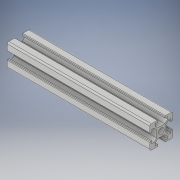
# Autodesk Inventor part: 2020-125mm
Saved by Autodesk Inventor 2019 (Build 230136000, 136)
## iProperties
Created: 2019-04-21
Part Number: 2020-125mm
Material: Generic
Document SubType Name: Modeling
Designer: Alex Jones
Density: 1 g/cm^3
Appearance: Default
Author: Alex Jones
Autodesk Inventor part; units mm, degrees
ref_plane "YZ Plane" through (0, 0, 0) normal (1, 0, 0) x (0, 1, 0)
ref_plane "XZ Plane" through (0, 0, 0) normal (0, 1, 0) x (-1, 0, 0)
ref_plane "XY Plane" through (0, 0, 0) normal (0, 0, 1) x (1, 0, 0)
sketch "Sketch1" plane through (0, 0, 0) normal (1, 0, 0) x (0, 1, 0)
  circle A0 centre (0, 0) radius 2.5
  line L0 (0, 0) -> (10, 0)
  line L1 (10, -10) -> (10, -3.6)
  line L2 (10, -3.6) -> (9.5, -3.1)
  line L3 (9.5, -3.1) -> (8.4, -3.1)
  line L4 (8.4, -3.1) -> (8.4, -5.5)
  line L5 (-3.134, 4.1) -> (3.134, 4.1)
  line L6 (4.1, 3.134) -> (4.1, -3.134)
  line L7 (3.134, -4.1) -> (-3.134, -4.1)
  line L8 (-4.1, -3.134) -> (-4.1, 3.134)
  line L9 (-4.1, 4.1) -> (4.1, -4.1) construction
  line L10 (4.1, 4.1) -> (-4.1, -4.1) construction
  line L11 (4.1, -3.134) -> (6.466, -5.5)
  line L12 (8.4, -5.5) -> (6.466, -5.5)
  line L13 (10, -10) -> (3.6, -10)
  line L14 (3.6, -10) -> (3.1, -9.5)
  line L15 (3.1, -9.5) -> (3.1, -8.4)
  line L16 (3.1, -8.4) -> (5.5, -8.4)
  line L17 (3.134, -4.1) -> (5.5, -6.466)
  line L18 (5.5, -8.4) -> (5.5, -6.466)
  line L19 (10, 10) -> (10, 3.6)
  line L20 (10, 3.6) -> (9.5, 3.1)
  line L21 (9.5, 3.1) -> (8.4, 3.1)
  line L22 (8.4, 3.1) -> (8.4, 5.5)
  line L23 (4.1, 3.134) -> (6.466, 5.5)
  line L24 (8.4, 5.5) -> (6.466, 5.5)
  line L25 (5.5, 8.4) -> (5.5, 6.466)
  line L26 (3.134, 4.1) -> (5.5, 6.466)
  line L27 (3.1, 8.4) -> (5.5, 8.4)
  line L28 (3.1, 9.5) -> (3.1, 8.4)
  line L29 (3.6, 10) -> (3.1, 9.5)
  line L30 (10, 10) -> (3.6, 10)
  line L31 (0, 0) -> (0, -5.5)
  line L32 (-10, -10) -> (-10, -3.6)
  line L33 (-10, -3.6) -> (-9.5, -3.1)
  line L34 (-9.5, -3.1) -> (-8.4, -3.1)
  line L35 (-8.4, -3.1) -> (-8.4, -5.5)
  line L36 (-4.1, -3.134) -> (-6.466, -5.5)
  line L37 (-8.4, -5.5) -> (-6.466, -5.5)
  line L38 (-5.5, -8.4) -> (-5.5, -6.466)
  line L39 (-3.134, -4.1) -> (-5.5, -6.466)
  line L40 (-3.1, -8.4) -> (-5.5, -8.4)
  line L41 (-3.1, -9.5) -> (-3.1, -8.4)
  line L42 (-3.6, -10) -> (-3.1, -9.5)
  line L43 (-10, -10) -> (-3.6, -10)
  line L44 (-4.1, 3.134) -> (-6.466, 5.5)
  line L45 (-3.134, 4.1) -> (-5.5, 6.466)
  line L46 (-8.4, 3.1) -> (-8.4, 5.5)
  line L47 (-8.4, 5.5) -> (-6.466, 5.5)
  line L48 (-5.5, 8.4) -> (-5.5, 6.466)
  line L49 (-3.1, 8.4) -> (-5.5, 8.4)
  line L50 (-9.5, 3.1) -> (-8.4, 3.1)
  line L51 (-10, 3.6) -> (-9.5, 3.1)
  line L52 (-3.1, 9.5) -> (-3.1, 8.4)
  line L53 (-3.6, 10) -> (-3.1, 9.5)
  line L54 (-10, 10) -> (-3.6, 10)
  line L55 (-10, 10) -> (-10, 3.6)
  point P0 (-10, 0)
  dimension "d0" = 5
  dimension "d3" = 3.6
  dimension "d4" = 45
  dimension "d5" = 3.1
  dimension "d7" = 5.5
  dimension "d8" = 1.6
  dimension "d11" = 4.3
  constraints: 112 end point, 40 symmetric about line, 4 horizontal, 3 vertical, 2 midpoint, 2 parallel, 1 centre point, 1 coincident, 1 perpendicular
  measures "d0" diameter of A0
  measures "d3" distance of L0.end L1.end
  measures "d4" angle of L0 L2
  measures "d5" distance from line of L0 L2.end
  measures "d7" distance from line of L0 L4.end
  measures "d8" distance between parallel lines of L1 L4
  measures "d11" distance between parallel lines of L6 L4
extrude "Extrusion1" add sketch "Sketch1" along normal blind 125 contours L0 L6 L11 L12 L4 L3 L2 L1 L13 L14 L15 L16 L18 L17 L7 L31 A0 | A0 L31 L7 L39 L38 L40 L41 L42 L43 L32 L33 L34 L35 L37 L36 L8 L44 L47 L46 L50 L51 L55 L54 L53 L52 L49 L48 L45 L5 L26 L25 L27 L28 L29 L30 L19 L20 L21 L22 L24 L23 L6 L0
fillet "Fillet1" radius 1.25 4 edges at (62.5, 10, 10) (62.5, -10, 10) (62.5, 10, -10) (62.5, -10, -10)
body "Solid1"
